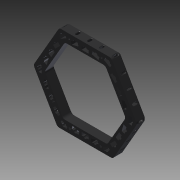
# Autodesk Inventor part: TSOP Cover Ring
Saved by Autodesk Inventor 2015 (Build 190159000, 159)
## iProperties
Created: 2016-10-13
Part Number: TSOP Cover Ring
Material: Generic
Document SubType Name: Modeling
Designer: James Yelland
Density: 1 g/cm^3
Appearance: Default
Author: James Yelland
Autodesk Inventor part; units mm, degrees
ref_plane "YZ Plane" through (0, 0, 0) normal (1, 0, 0) x (0, 1, 0)
ref_plane "XZ Plane" through (0, 0, 0) normal (0, 1, 0) x (-1, 0, 0)
ref_plane "XY Plane" through (0, 0, 0) normal (0, 0, 1) x (1, 0, 0)
sketch "Sketch1" plane through (0, 0, 0) normal (0, 1, 0) x (-1, 0, 0)
  circle A0 centre (24, -57.282) radius 1.6
  circle A1 centre (-25, 62.282) radius 1.6
  circle A2 centre (25, 62.282) radius 1.6
  circle A3 centre (-24, -57.282) radius 1.6
  line L0 (-40, -64.282) -> (40, -64.282)
  arc A4 (40, -64.282) -> (44.3301, -61.782) centre (40, -59.282) ccw
  line L1 (44.3301, -61.782) -> (78.5566, -2.5)
  arc A5 (78.5566, -2.5) -> (78.5566, 2.5) centre (74.2265, 0) ccw
  line L2 (78.5566, 2.5) -> (41.4434, 66.782)
  arc A6 (41.4434, 66.782) -> (37.1132, 69.282) centre (37.1132, 64.282) ccw
  line L3 (37.1132, 69.282) -> (-37.1132, 69.282)
  arc A7 (-37.1132, 69.282) -> (-41.4434, 66.782) centre (-37.1132, 64.282) ccw
  line L4 (-41.4434, 66.782) -> (-78.5566, 2.5)
  arc A8 (-78.5566, 2.5) -> (-78.5566, -2.5) centre (-74.2265, 0) ccw
  line L5 (-78.5566, -2.5) -> (-44.3301, -61.782)
  arc A9 (-44.3301, -61.782) -> (-40, -64.282) centre (-40, -59.282) ccw
  line L6 (47.0096, -27.141) -> (35.6699, -46.782)
  line L7 (0, -49.282) -> (-31.3397, -49.282)
  line L8 (-47.0096, -27.141) -> (-61.2361, -2.5)
  line L9 (-47.0096, 27.141) -> (-32.7831, 51.782)
  line L10 (47.0096, 27.141) -> (32.7831, 51.782)
  line L11 (47.0096, 27.141) -> (61.2361, 2.5)
  line L12 (28.453, 54.282) -> (0, 54.282)
  line L13 (0, 54.282) -> (-28.453, 54.282)
  line L14 (61.2361, -2.5) -> (47.0096, -27.141)
  line L15 (31.3397, -49.282) -> (0, -49.282)
  line L16 (-35.6699, -46.782) -> (-47.0096, -27.141)
  line L17 (-47.0096, 27.141) -> (-61.2361, 2.5)
  arc A10 (31.3397, -49.282) -> (35.6699, -46.782) centre (31.3397, -44.282) ccw
  arc A11 (-35.6699, -46.782) -> (-31.3397, -49.282) centre (-31.3397, -44.282) ccw
  arc A12 (-61.2361, 2.5) -> (-61.2361, -2.5) centre (-56.906, 0) ccw
  arc A13 (-28.453, 54.282) -> (-32.7831, 51.782) centre (-28.453, 49.282) ccw
  arc A14 (32.7831, 51.782) -> (28.453, 54.282) centre (28.453, 49.282) ccw
  arc A15 (61.2361, -2.5) -> (61.2361, 2.5) centre (56.906, 0) ccw
  line L18 (-52.4809, 24.0645) -> (-47.0809, 33.4176)
  arc A16 (-52.6475, 33.376) -> (-55.2282, 28.9061) centre (-53.1151, 30.666) ccw
  line L19 (-56.6378, 26.4645) -> (-55.2282, 28.9061)
  line L20 (-56.6378, 26.4645) -> (-52.4809, 24.0645)
  line L21 (-47.0809, 33.4176) -> (-51.2378, 35.8176)
  line L22 (-52.6475, 33.376) -> (-51.2378, 35.8176)
  line L23 (-56.4865, 20.726) -> (-61.1229, 21.9683)
  line L24 (-61.8526, 19.2451) -> (-61.1229, 21.9683)
  arc A17 (-61.8526, 19.2451) -> (-63.1885, 14.2596) centre (-61.6029, 16.5065) ccw
  line L25 (-59.2817, 10.294) -> (-56.4865, 20.726)
  line L26 (-63.9182, 11.5363) -> (-63.1885, 14.2596)
  line L27 (-63.9182, 11.5363) -> (-59.2817, 10.294)
  line L28 (-67.4265, 5.4) -> (-72.2265, 5.4)
  line L29 (-72.2265, 2.5807) -> (-72.2265, 5.4)
  arc A18 (-72.2265, 2.5807) -> (-72.2265, -2.5807) centre (-71.2765, 0) ccw
  line L30 (-67.4265, -5.4) -> (-67.4265, 5.4)
  line L31 (-72.2265, -5.4) -> (-72.2265, -2.5807)
  line L32 (-72.2265, -5.4) -> (-67.4265, -5.4)
  line L33 (-59.2817, -10.294) -> (-63.9182, -11.5363)
  line L34 (-63.1885, -14.2596) -> (-63.9182, -11.5363)
  arc A19 (-63.1885, -14.2596) -> (-61.8526, -19.2451) centre (-61.6029, -16.5065) ccw
  line L35 (-56.4865, -20.726) -> (-59.2817, -10.294)
  line L36 (-61.1229, -21.9683) -> (-61.8526, -19.2451)
  line L37 (-61.1229, -21.9683) -> (-56.4865, -20.726)
  line L38 (-52.4809, -24.0645) -> (-56.6378, -26.4645)
  line L39 (-55.2282, -28.9061) -> (-56.6378, -26.4645)
  arc A20 (-55.2282, -28.9061) -> (-52.6475, -33.376) centre (-53.1151, -30.666) ccw
  line L40 (-47.0809, -33.4176) -> (-52.4809, -24.0645)
  line L41 (-51.2378, -35.8176) -> (-52.6475, -33.376)
  line L42 (-51.2378, -35.8176) -> (-47.0809, -33.4176)
  line L43 (-46.1925, -38.5557) -> (-49.5866, -41.9498)
  line L44 (-47.593, -43.9434) -> (-49.5866, -41.9498)
  arc A21 (-47.593, -43.9434) -> (-43.9434, -47.593) centre (-45.0965, -45.0965) ccw
  line L45 (-38.5557, -46.1925) -> (-46.1925, -38.5557)
  line L46 (-41.9498, -49.5866) -> (-43.9434, -47.593)
  line L47 (-41.9498, -49.5866) -> (-38.5557, -46.1925)
  line L48 (-35.8898, -51.3629) -> (-38.2898, -55.5199)
  line L49 (-35.8482, -56.9295) -> (-38.2898, -55.5199)
  arc A22 (-35.8482, -56.9295) -> (-31.3783, -59.5102) centre (-33.1382, -57.3971) ccw
  line L50 (-26.5367, -56.7629) -> (-35.8898, -51.3629)
  line L51 (-28.9367, -60.9199) -> (-31.3783, -59.5102)
  line L52 (-28.9367, -60.9199) -> (-26.5367, -56.7629)
  line L53 (-19.3863, -51.4865) -> (-20.6286, -56.1229)
  line L54 (-17.9053, -56.8526) -> (-20.6286, -56.1229)
  arc A23 (-17.9053, -56.8526) -> (-12.9198, -58.1885) centre (-15.1667, -56.6029) ccw
  line L55 (-8.9543, -54.2817) -> (-19.3863, -51.4865)
  line L56 (-10.1966, -58.9182) -> (-12.9198, -58.1885)
  line L57 (-10.1966, -58.9182) -> (-8.9543, -54.2817)
  line L58 (-5.4, -52.482) -> (-5.4, -57.282)
  line L59 (-2.5807, -57.282) -> (-5.4, -57.282)
  arc A24 (-2.5807, -57.282) -> (2.5807, -57.282) centre (0, -56.332) ccw
  line L60 (5.4, -52.482) -> (-5.4, -52.482)
  line L61 (5.4, -57.282) -> (2.5807, -57.282)
  line L62 (5.4, -57.282) -> (5.4, -52.482)
  line L63 (8.9543, -54.2817) -> (10.1966, -58.9182)
  line L64 (12.9198, -58.1885) -> (10.1966, -58.9182)
  arc A25 (12.9198, -58.1885) -> (17.9053, -56.8526) centre (15.1667, -56.6029) ccw
  line L65 (19.3863, -51.4865) -> (8.9543, -54.2817)
  line L66 (20.6286, -56.1229) -> (17.9053, -56.8526)
  line L67 (20.6286, -56.1229) -> (19.3863, -51.4865)
  line L68 (-205.3728, -147.5875) -> (-202.9728, -151.7445)
  line L69 (-200.5312, -150.3348) -> (-202.9728, -151.7445)
  line L70 (-197.3963, -150.6033) -> (-198.7713, -148.2217)
  arc A26 (-200.5312, -150.3348) -> (-196.0613, -147.7541) centre (-198.7713, -148.2217) ccw
  line L71 (-196.0197, -142.1875) -> (-205.3728, -147.5875)
  line L72 (-193.6197, -146.3445) -> (-196.0613, -147.7541)
  line L73 (-193.6197, -146.3445) -> (-196.0197, -142.1875)
  line L74 (38.5557, -46.1925) -> (41.9498, -49.5866)
  line L75 (43.9434, -47.593) -> (41.9498, -49.5866)
  arc A27 (43.9434, -47.593) -> (47.593, -43.9434) centre (45.0965, -45.0965) ccw
  line L76 (46.1925, -38.5557) -> (38.5557, -46.1925)
  line L77 (49.5866, -41.9498) -> (47.593, -43.9434)
  line L78 (49.5866, -41.9498) -> (46.1925, -38.5557)
  line L79 (47.0809, -33.4176) -> (51.2378, -35.8176)
  line L80 (52.6475, -33.376) -> (51.2378, -35.8176)
  arc A28 (52.6475, -33.376) -> (55.2282, -28.9061) centre (53.1151, -30.666) ccw
  line L81 (52.4809, -24.0645) -> (47.0809, -33.4176)
  line L82 (56.6378, -26.4645) -> (55.2282, -28.9061)
  line L83 (56.6378, -26.4645) -> (52.4809, -24.0645)
  line L84 (56.4865, -20.726) -> (61.1229, -21.9683)
  line L85 (61.8526, -19.2451) -> (61.1229, -21.9683)
  arc A29 (61.8526, -19.2451) -> (63.1885, -14.2596) centre (61.6029, -16.5065) ccw
  line L86 (59.2817, -10.294) -> (56.4865, -20.726)
  line L87 (63.9182, -11.5363) -> (63.1885, -14.2596)
  line L88 (63.9182, -11.5363) -> (59.2817, -10.294)
  line L89 (67.4265, -5.4) -> (72.2265, -5.4)
  line L90 (72.2265, -2.5807) -> (72.2265, -5.4)
  arc A30 (72.2265, -2.5807) -> (72.2265, 2.5807) centre (71.2765, 0) ccw
  line L91 (67.4265, 5.4) -> (67.4265, -5.4)
  line L92 (72.2265, 5.4) -> (72.2265, 2.5807)
  line L93 (72.2265, 5.4) -> (67.4265, 5.4)
  line L94 (59.2817, 10.294) -> (63.9182, 11.5363)
  line L95 (63.1885, 14.2596) -> (63.9182, 11.5363)
  arc A31 (63.1885, 14.2596) -> (61.8526, 19.2451) centre (61.6029, 16.5065) ccw
  line L96 (56.4865, 20.726) -> (59.2817, 10.294)
  line L97 (61.1229, 21.9683) -> (61.8526, 19.2451)
  line L98 (61.1229, 21.9683) -> (56.4865, 20.726)
  line L99 (52.4809, 24.0645) -> (56.6378, 26.4645)
  line L100 (55.2282, 28.9061) -> (56.6378, 26.4645)
  arc A32 (55.2282, 28.9061) -> (52.6475, 33.376) centre (53.1151, 30.666) ccw
  line L101 (47.0809, 33.4176) -> (52.4809, 24.0645)
  line L102 (51.2378, 35.8176) -> (52.6475, 33.376)
  line L103 (51.2378, 35.8176) -> (47.0809, 33.4176)
  line L104 (46.1925, 38.5557) -> (49.5866, 41.9498)
  line L105 (47.593, 43.9434) -> (49.5866, 41.9498)
  arc A33 (47.593, 43.9434) -> (43.9434, 47.593) centre (45.0965, 45.0965) ccw
  line L106 (38.5557, 46.1925) -> (46.1925, 38.5557)
  line L107 (41.9498, 49.5866) -> (43.9434, 47.593)
  line L108 (41.9498, 49.5866) -> (38.5557, 46.1925)
  line L109 (38.3898, 55.6931) -> (40.7898, 59.85)
  line L110 (38.3482, 61.2596) -> (40.7898, 59.85)
  arc A34 (38.3482, 61.2596) -> (33.8783, 63.8403) centre (35.6382, 61.7273) ccw
  line L111 (29.0367, 61.0931) -> (38.3898, 55.6931)
  line L112 (31.4367, 65.25) -> (33.8783, 63.8403)
  line L113 (31.4367, 65.25) -> (29.0367, 61.0931)
  line L114 (20.726, 56.4865) -> (21.9683, 61.1229)
  line L115 (19.2451, 61.8526) -> (21.9683, 61.1229)
  arc A35 (19.2451, 61.8526) -> (14.2596, 63.1885) centre (16.5065, 61.6029) ccw
  line L116 (10.294, 59.2817) -> (20.726, 56.4865)
  line L117 (11.5363, 63.9182) -> (14.2596, 63.1885)
  line L118 (11.5363, 63.9182) -> (10.294, 59.2817)
  line L119 (5.4, 57.482) -> (5.4, 62.282)
  line L120 (2.5807, 62.282) -> (5.4, 62.282)
  arc A36 (2.5807, 62.282) -> (-2.5807, 62.282) centre (0, 61.332) ccw
  line L121 (-5.4, 57.482) -> (5.4, 57.482)
  line L122 (-5.4, 62.282) -> (-2.5807, 62.282)
  line L123 (-5.4, 62.282) -> (-5.4, 57.482)
  line L124 (-10.294, 59.2817) -> (-11.5363, 63.9182)
  line L125 (-14.2596, 63.1885) -> (-11.5363, 63.9182)
  arc A37 (-14.2596, 63.1885) -> (-19.2451, 61.8526) centre (-16.5065, 61.6029) ccw
  line L126 (-20.726, 56.4865) -> (-10.294, 59.2817)
  line L127 (-21.9683, 61.1229) -> (-19.2451, 61.8526)
  line L128 (-21.9683, 61.1229) -> (-20.726, 56.4865)
  line L129 (-29.0367, 61.0931) -> (-31.4367, 65.25)
  line L130 (-33.8783, 63.8403) -> (-31.4367, 65.25)
  arc A38 (-33.8783, 63.8403) -> (-38.3482, 61.2596) centre (-35.6382, 61.7273) ccw
  line L131 (-38.3898, 55.6931) -> (-29.0367, 61.0931)
  line L132 (-40.7898, 59.85) -> (-38.3482, 61.2596)
  line L133 (-40.7898, 59.85) -> (-38.3898, 55.6931)
  line L134 (-38.5557, 46.1925) -> (-41.9498, 49.5866)
  line L135 (-43.9434, 47.593) -> (-41.9498, 49.5866)
  arc A39 (-43.9434, 47.593) -> (-47.593, 43.9434) centre (-45.0965, 45.0965) ccw
  line L136 (-46.1925, 38.5557) -> (-38.5557, 46.1925)
  line L137 (-49.5866, 41.9498) -> (-47.593, 43.9434)
  line L138 (-49.5866, 41.9498) -> (-46.1925, 38.5557)
  line L139 (37.9434, -55.7199) -> (35.8482, -56.9295)
  arc A40 (31.3783, -59.5102) -> (35.8482, -56.9295) centre (33.1382, -57.3971) ccw
  line L140 (31.3783, -59.5102) -> (29.2831, -60.7199)
  line L141 (29.2831, -60.7199) -> (27.2831, -57.2558)
  line L142 (27.2831, -57.2558) -> (35.9434, -52.2558)
  line L143 (35.9434, -52.2558) -> (37.9434, -55.7199)
  constraints: 288 end point, 74 point on circle, 52 centre point, 12 tangent, 5 equal radius, 4 horizontal
extrude "Extrusion1" add sketch "Sketch1" along normal blind 15 contours A9 L5 A8 L4 A7 L3 A6 L2 A5 L1 A4 L0
sketch "Sketch2" plane through (0, 15, 0) normal (0, 1, 0) x (1, 0, 0)
  arc A0 (35.6699, 46.782) -> (31.3397, 49.282) centre (31.3397, 44.282) ccw projected
  line L0 (35.6699, 46.782) -> (61.2361, 2.5) projected
  arc A1 (61.2361, -2.5) -> (61.2361, 2.5) centre (56.906, 0) ccw projected
  line L1 (61.2361, -2.5) -> (32.7831, -51.782) projected
  arc A2 (28.453, -54.282) -> (32.7831, -51.782) centre (28.453, -49.282) ccw projected
  line L2 (28.453, -54.282) -> (-28.453, -54.282) projected
  arc A3 (-32.7831, -51.782) -> (-28.453, -54.282) centre (-28.453, -49.282) ccw projected
  line L3 (-32.7831, -51.782) -> (-61.2361, -2.5) projected
  arc A4 (-61.2361, 2.5) -> (-61.2361, -2.5) centre (-56.906, 0) ccw projected
  line L4 (-61.2361, 2.5) -> (-35.6699, 46.782) projected
  arc A5 (-31.3397, 49.282) -> (-35.6699, 46.782) centre (-31.3397, 44.282) ccw projected
  line L5 (-31.3397, 49.282) -> (31.3397, 49.282) projected
  line L6 (38.5557, -46.1925) -> (46.1925, -38.5557) projected
  line L7 (46.1925, -38.5557) -> (49.5866, -41.9498) projected
  line L8 (49.5866, -41.9498) -> (47.593, -43.9434) projected
  arc A6 (43.9434, -47.593) -> (47.593, -43.9434) centre (45.0965, -45.0965) ccw projected
  line L9 (43.9434, -47.593) -> (41.9498, -49.5866) projected
  line L10 (41.9498, -49.5866) -> (38.5557, -46.1925) projected
  line L11 (29.0367, -61.0931) -> (38.3898, -55.6931) projected
  line L12 (38.3898, -55.6931) -> (40.7898, -59.85) projected
  line L13 (40.7898, -59.85) -> (38.3482, -61.2596) projected
  arc A7 (33.8783, -63.8403) -> (38.3482, -61.2596) centre (35.6382, -61.7273) ccw projected
  line L14 (33.8783, -63.8403) -> (31.4367, -65.25) projected
  line L15 (31.4367, -65.25) -> (29.0367, -61.0931) projected
  line L16 (10.294, -59.2817) -> (20.726, -56.4865) projected
  line L17 (20.726, -56.4865) -> (21.9683, -61.1229) projected
  line L18 (21.9683, -61.1229) -> (19.2451, -61.8526) projected
  arc A8 (14.2596, -63.1885) -> (19.2451, -61.8526) centre (16.5065, -61.6029) ccw projected
  line L19 (14.2596, -63.1885) -> (11.5363, -63.9182) projected
  line L20 (11.5363, -63.9182) -> (10.294, -59.2817) projected
  line L21 (-5.4, -57.482) -> (5.4, -57.482) projected
  line L22 (5.4, -57.482) -> (5.4, -62.282) projected
  line L23 (5.4, -62.282) -> (2.5807, -62.282) projected
  arc A9 (-2.5807, -62.282) -> (2.5807, -62.282) centre (0, -61.332) ccw projected
  line L24 (-2.5807, -62.282) -> (-5.4, -62.282) projected
  line L25 (-5.4, -62.282) -> (-5.4, -57.482) projected
  line L26 (-20.726, -56.4865) -> (-10.294, -59.2817) projected
  line L27 (-10.294, -59.2817) -> (-11.5363, -63.9182) projected
  line L28 (-11.5363, -63.9182) -> (-14.2596, -63.1885) projected
  arc A10 (-19.2451, -61.8526) -> (-14.2596, -63.1885) centre (-16.5065, -61.6029) ccw projected
  line L29 (-19.2451, -61.8526) -> (-21.9683, -61.1229) projected
  line L30 (-21.9683, -61.1229) -> (-20.726, -56.4865) projected
  line L31 (-38.3898, -55.6931) -> (-29.0367, -61.0931) projected
  line L32 (-29.0367, -61.0931) -> (-31.4367, -65.25) projected
  line L33 (-31.4367, -65.25) -> (-33.8783, -63.8403) projected
  arc A11 (-38.3482, -61.2596) -> (-33.8783, -63.8403) centre (-35.6382, -61.7273) ccw projected
  line L34 (-38.3482, -61.2596) -> (-40.7898, -59.85) projected
  line L35 (-40.7898, -59.85) -> (-38.3898, -55.6931) projected
  line L36 (-46.1925, -38.5557) -> (-38.5557, -46.1925) projected
  line L37 (-38.5557, -46.1925) -> (-41.9498, -49.5866) projected
  line L38 (-41.9498, -49.5866) -> (-43.9434, -47.593) projected
  arc A12 (-47.593, -43.9434) -> (-43.9434, -47.593) centre (-45.0965, -45.0965) ccw projected
  line L39 (-47.593, -43.9434) -> (-49.5866, -41.9498) projected
  line L40 (-49.5866, -41.9498) -> (-46.1925, -38.5557) projected
  line L41 (-52.4809, -24.0645) -> (-47.0809, -33.4176) projected
  line L42 (-47.0809, -33.4176) -> (-51.2378, -35.8176) projected
  line L43 (-51.2378, -35.8176) -> (-52.6475, -33.376) projected
  arc A13 (-55.2282, -28.9061) -> (-52.6475, -33.376) centre (-53.1151, -30.666) ccw projected
  line L44 (-55.2282, -28.9061) -> (-56.6378, -26.4645) projected
  line L45 (-56.6378, -26.4645) -> (-52.4809, -24.0645) projected
  line L46 (-59.2817, -10.294) -> (-56.4865, -20.726) projected
  line L47 (-56.4865, -20.726) -> (-61.1229, -21.9683) projected
  line L48 (-61.1229, -21.9683) -> (-61.8526, -19.2451) projected
  arc A14 (-63.1885, -14.2596) -> (-61.8526, -19.2451) centre (-61.6029, -16.5065) ccw projected
  line L49 (-63.1885, -14.2596) -> (-63.9182, -11.5363) projected
  line L50 (-63.9182, -11.5363) -> (-59.2817, -10.294) projected
  line L51 (-67.4265, 5.4) -> (-67.4265, -5.4) projected
  line L52 (-67.4265, -5.4) -> (-72.2265, -5.4) projected
  line L53 (-72.2265, -5.4) -> (-72.2265, -2.5807) projected
  arc A15 (-72.2265, 2.5807) -> (-72.2265, -2.5807) centre (-71.2765, 0) ccw projected
  line L54 (-72.2265, 2.5807) -> (-72.2265, 5.4) projected
  line L55 (-72.2265, 5.4) -> (-67.4265, 5.4) projected
  line L56 (-56.4865, 20.726) -> (-59.2817, 10.294) projected
  line L57 (-59.2817, 10.294) -> (-63.9182, 11.5363) projected
  line L58 (-63.9182, 11.5363) -> (-63.1885, 14.2596) projected
  arc A16 (-61.8526, 19.2451) -> (-63.1885, 14.2596) centre (-61.6029, 16.5065) ccw projected
  line L59 (-61.8526, 19.2451) -> (-61.1229, 21.9683) projected
  line L60 (-61.1229, 21.9683) -> (-56.4865, 20.726) projected
  line L61 (-47.0809, 33.4176) -> (-52.4809, 24.0645) projected
  line L62 (-52.4809, 24.0645) -> (-56.6378, 26.4645) projected
  line L63 (-56.6378, 26.4645) -> (-55.2282, 28.9061) projected
  arc A17 (-52.6475, 33.376) -> (-55.2282, 28.9061) centre (-53.1151, 30.666) ccw projected
  line L64 (-52.6475, 33.376) -> (-51.2378, 35.8176) projected
  line L65 (-51.2378, 35.8176) -> (-47.0809, 33.4176) projected
  line L66 (-38.5557, 46.1925) -> (-46.1925, 38.5557) projected
  line L67 (-46.1925, 38.5557) -> (-49.5866, 41.9498) projected
  line L68 (-49.5866, 41.9498) -> (-47.593, 43.9434) projected
  arc A18 (-43.9434, 47.593) -> (-47.593, 43.9434) centre (-45.0965, 45.0965) ccw projected
  line L69 (-43.9434, 47.593) -> (-41.9498, 49.5866) projected
  line L70 (-41.9498, 49.5866) -> (-38.5557, 46.1925) projected
  line L71 (-8.9543, 54.2817) -> (-19.3863, 51.4865) projected
  line L72 (-19.3863, 51.4865) -> (-20.6286, 56.1229) projected
  line L73 (-20.6286, 56.1229) -> (-17.9053, 56.8526) projected
  arc A19 (-12.9198, 58.1885) -> (-17.9053, 56.8526) centre (-15.1667, 56.6029) ccw projected
  line L74 (-12.9198, 58.1885) -> (-10.1966, 58.9182) projected
  line L75 (-10.1966, 58.9182) -> (-8.9543, 54.2817) projected
  line L76 (5.4, 52.482) -> (-5.4, 52.482) projected
  line L77 (-5.4, 52.482) -> (-5.4, 57.282) projected
  line L78 (-5.4, 57.282) -> (-2.5807, 57.282) projected
  arc A20 (2.5807, 57.282) -> (-2.5807, 57.282) centre (0, 56.332) ccw projected
  line L79 (2.5807, 57.282) -> (5.4, 57.282) projected
  line L80 (5.4, 57.282) -> (5.4, 52.482) projected
  line L81 (19.3863, 51.4865) -> (8.9543, 54.2817) projected
  line L82 (8.9543, 54.2817) -> (10.1966, 58.9182) projected
  line L83 (10.1966, 58.9182) -> (12.9198, 58.1885) projected
  arc A21 (17.9053, 56.8526) -> (12.9198, 58.1885) centre (15.1667, 56.6029) ccw projected
  line L84 (17.9053, 56.8526) -> (20.6286, 56.1229) projected
  line L85 (20.6286, 56.1229) -> (19.3863, 51.4865) projected
  line L86 (35.8898, 51.3629) -> (26.5367, 56.7629) projected
  line L87 (26.5367, 56.7629) -> (28.9367, 60.9199) projected
  line L88 (28.9367, 60.9199) -> (31.3783, 59.5102) projected
  arc A22 (35.8482, 56.9295) -> (31.3783, 59.5102) centre (33.1382, 57.3971) ccw projected
  line L89 (35.8482, 56.9295) -> (38.2898, 55.5199) projected
  line L90 (38.2898, 55.5199) -> (35.8898, 51.3629) projected
  line L91 (46.1925, 38.5557) -> (38.5557, 46.1925) projected
  line L92 (38.5557, 46.1925) -> (41.9498, 49.5866) projected
  line L93 (41.9498, 49.5866) -> (43.9434, 47.593) projected
  arc A23 (47.593, 43.9434) -> (43.9434, 47.593) centre (45.0965, 45.0965) ccw projected
  line L94 (47.593, 43.9434) -> (49.5866, 41.9498) projected
  line L95 (49.5866, 41.9498) -> (46.1925, 38.5557) projected
  line L96 (52.4809, 24.0645) -> (47.0809, 33.4176) projected
  line L97 (47.0809, 33.4176) -> (51.2378, 35.8176) projected
  line L98 (51.2378, 35.8176) -> (52.6475, 33.376) projected
  arc A24 (55.2282, 28.9061) -> (52.6475, 33.376) centre (53.1151, 30.666) ccw projected
  line L99 (55.2282, 28.9061) -> (56.6378, 26.4645) projected
  line L100 (56.6378, 26.4645) -> (52.4809, 24.0645) projected
  line L101 (59.2817, 10.294) -> (56.4865, 20.726) projected
  line L102 (56.4865, 20.726) -> (61.1229, 21.9683) projected
  line L103 (61.1229, 21.9683) -> (61.8526, 19.2451) projected
  arc A25 (63.1885, 14.2596) -> (61.8526, 19.2451) centre (61.6029, 16.5065) ccw projected
  line L104 (63.1885, 14.2596) -> (63.9182, 11.5363) projected
  line L105 (63.9182, 11.5363) -> (59.2817, 10.294) projected
  line L106 (67.4265, -5.4) -> (67.4265, 5.4) projected
  line L107 (67.4265, 5.4) -> (72.2265, 5.4) projected
  line L108 (72.2265, 5.4) -> (72.2265, 2.5807) projected
  arc A26 (72.2265, -2.5807) -> (72.2265, 2.5807) centre (71.2765, 0) ccw projected
  line L109 (72.2265, -2.5807) -> (72.2265, -5.4) projected
  line L110 (72.2265, -5.4) -> (67.4265, -5.4) projected
  line L111 (56.4865, -20.726) -> (59.2817, -10.294) projected
  line L112 (59.2817, -10.294) -> (63.9182, -11.5363) projected
  line L113 (63.9182, -11.5363) -> (63.1885, -14.2596) projected
  arc A27 (61.8526, -19.2451) -> (63.1885, -14.2596) centre (61.6029, -16.5065) ccw projected
  line L114 (61.8526, -19.2451) -> (61.1229, -21.9683) projected
  line L115 (61.1229, -21.9683) -> (56.4865, -20.726) projected
  line L116 (52.4809, -24.0645) -> (56.6378, -26.4645) projected
  line L117 (56.6378, -26.4645) -> (55.2282, -28.9061) projected
  arc A28 (52.6475, -33.376) -> (55.2282, -28.9061) centre (53.1151, -30.666) ccw projected
  line L118 (52.6475, -33.376) -> (51.2378, -35.8176) projected
  line L119 (51.2378, -35.8176) -> (47.0809, -33.4176) projected
  line L120 (47.0809, -33.4176) -> (52.4809, -24.0645) projected
  line L121 (-27.2831, 57.2558) -> (-35.9434, 52.2558) projected
  line L122 (-35.9434, 52.2558) -> (-37.9434, 55.7199) projected
  line L123 (-37.9434, 55.7199) -> (-35.8482, 56.9295) projected
  arc A29 (-31.3783, 59.5102) -> (-35.8482, 56.9295) centre (-33.1382, 57.3971) ccw projected
  line L124 (-31.3783, 59.5102) -> (-29.2831, 60.7199) projected
  line L125 (-29.2831, 60.7199) -> (-27.2831, 57.2558) projected
  circle A30 centre (-25, -62.282) radius 1.6 projected
  circle A31 centre (24, 57.282) radius 1.6 projected
  circle A32 centre (25, -62.282) radius 1.6 projected
  circle A33 centre (-24, 57.282) radius 1.6 projected
  line L126 (40, 64.282) -> (-40, 64.282) projected
  arc A34 (-40, 64.282) -> (-44.3301, 61.782) centre (-40, 59.282) ccw projected
  line L127 (-44.3301, 61.782) -> (-78.5566, 2.5) projected
  arc A35 (-78.5566, 2.5) -> (-78.5566, -2.5) centre (-74.2265, 0) ccw projected
  line L128 (-78.5566, -2.5) -> (-41.4434, -66.782) projected
  arc A36 (-41.4434, -66.782) -> (-37.1132, -69.282) centre (-37.1132, -64.282) ccw projected
  line L129 (-37.1132, -69.282) -> (37.1132, -69.282) projected
  arc A37 (37.1132, -69.282) -> (41.4434, -66.782) centre (37.1132, -64.282) ccw projected
  line L130 (41.4434, -66.782) -> (78.5566, -2.5) projected
  arc A38 (78.5566, -2.5) -> (78.5566, 2.5) centre (74.2265, 0) ccw projected
  line L131 (78.5566, 2.5) -> (44.3301, 61.782) projected
  arc A39 (44.3301, 61.782) -> (40, 64.282) centre (40, 59.282) ccw projected
  point P0 (0, 0)
extrude "Extrusion2" add sketch "Sketch2" against normal blind 2 contours L6 L7 L8 A6 L9 L10 | L11 L12 L13 A7 L14 L15 | L16 L17 L18 A8 L19 L20 | L21 L22 L23 A9 L24 L25 | L26 L27 L28 A10 L29 L30 | L31 L32 L33 A11 L34 L35 | L36 L37 L38 A12 L39 L40 | L41 L42 L43 A13 L44 L45 | L46 L47 L48 A14 L49 L50 | L51 L52 L53 A15 L54 L55 | L56 L57 L58 A16 L59 L60 | L61 L62 L63 A17 L64 L65 | L66 L67 L68 A18 L69 L70 | L71 L72 L73 A19 L74 L75 | L76 L77 L78 A20 L79 L80 | L81 L82 L83 A21 L84 L85 | L86 L87 L88 A22 L89 L90 | L91 L92 L93 A23 L94 L95 | L96 L97 L98 A24 L99 L100 | L101 L102 L103 A25 L104 L105 | L106 L107 L108 A26 L109 L110 | L111 L112 L113 A27 L114 L115 | L116 L117 A28 L118 L119 L120 | L121 L122 L123 A29 L124 L125
chamfer "Chamfer1" distance 2 angle 45 12 edges at (0, 15, 69.282) (39.6132, 15, 68.6122) (60, 15, 34.641) (79.2265, 15, 0) (61.4434, 15, -32.141) (42.5, 15, -63.6122) (0, 15, -64.282) (-42.5, 15, -63.6122) (-61.4434, 15, -32.141) (-79.2265, 15, 0) (-60, 15, 34.641) (-39.6132, 15, 68.6122)
sketch "Sketch3" plane through (-47.0809, 0, -33.4176) normal (-0.8660254, 0, -0.5) x (-0.5, 0, 0.8660254)
  line L0 (5.4, 0) -> (5.4, 9.5)
  line L1 (3.9, 9.5) -> (3.9, 5.5)
  line L2 (6.9, 9.5) -> (6.9, 5.5)
  arc A0 (6.9, 9.5) -> (3.9, 9.5) centre (5.4, 9.5) ccw
  arc A1 (3.9, 5.5) -> (6.9, 5.5) centre (5.4, 5.5) ccw
  dimension "d27" = 9.5
  dimension "d29" = 4
  dimension "d30" = 4
  constraints: 6 end point, 4 point on circle, 3 vertical, 2 centre point, 1 coincident, 1 point on line
  measures "d27" distance of L0.start L0.end
  measures "d29" distance of L1.start L1.end
  measures "d30" distance of L2.start L2.end
extrude "Extrusion3" cut sketch "Sketch3" along normal through all
pattern_circular "Circular Pattern1" count 5 over 240 about axis through (0, -10, 0) along (0, 1, 0) of "Extrusion3"
sketch "Sketch4" plane through (46.1925, 0, -38.5557) normal (0.7071068, 0, -0.7071068) x (-0.7071068, 0, -0.7071068)
  line L0 (5.4, 0) -> (5.4, 9.5)
  line L1 (3.9, 9.5) -> (3.9, 5.5)
  line L2 (6.9, 9.5) -> (6.9, 5.5)
  arc A0 (6.9, 9.5) -> (3.9, 9.5) centre (5.4, 9.5) ccw
  arc A1 (3.9, 5.5) -> (6.9, 5.5) centre (5.4, 5.5) ccw
  point P0 (5.4, 0)
  dimension "d39" = 9.5
  dimension "d40" = 4
  dimension "d41" = 4
  constraints: 6 end point, 4 point on circle, 3 vertical, 2 centre point, 1 coincident, 1 point on line
  measures "d39" distance of L0.start L0.end
  measures "d40" distance of L1.start L1.end
  measures "d41" distance of L2.start L2.end
extrude "Extrusion4" cut sketch "Sketch4" along normal through all
pattern_circular "Circular Pattern2" count 5 over 240 about axis through (0, -10, 0) along (0, -1, 0) of "Extrusion4"
sketch "Sketch5" plane through (59.2817, 0, -10.294) normal (0.9659258, 0, -0.258819) x (-0.258819, 0, -0.9659258)
  line L0 (5.4, 0) -> (5.4, 9.5)
  line L1 (3.9, 9.5) -> (3.9, 5.5)
  line L2 (6.9, 9.5) -> (6.9, 5.5)
  arc A0 (6.9, 9.5) -> (3.9, 9.5) centre (5.4, 9.5) ccw
  arc A1 (3.9, 5.5) -> (6.9, 5.5) centre (5.4, 5.5) ccw
  point P0 (5.4, 0)
  dimension "d47" = 9.5
  dimension "d48" = 4
  dimension "d49" = 4
  constraints: 6 end point, 4 point on circle, 3 vertical, 2 centre point, 1 coincident, 1 point on line
  measures "d47" distance of L0.start L0.end
  measures "d48" distance of L1.start L1.end
  measures "d49" distance of L2.start L2.end
extrude "Extrusion5" cut sketch "Sketch5" along normal through all
pattern_circular "Circular Pattern3" count 5 over 240 about axis through (0, -10, 0) along (0, -1, 0) of "Extrusion5"
sketch "Sketch6" plane through (67.4265, 0, 5.4) normal (1, 0, 0) x (0, 0, -1)
  line L0 (5.4, 0) -> (5.4, 9.5)
  line L1 (3.9, 9.5) -> (3.9, 5.5)
  line L2 (6.9, 9.5) -> (6.9, 5.5)
  arc A0 (6.9, 9.5) -> (3.9, 9.5) centre (5.4, 9.5) ccw
  arc A1 (3.9, 5.5) -> (6.9, 5.5) centre (5.4, 5.5) ccw
  point P0 (5.4, 0)
  dimension "d55" = 9.5
  dimension "d56" = 4
  dimension "d57" = 4
  constraints: 6 end point, 4 point on circle, 3 vertical, 2 centre point, 1 coincident, 1 point on line
  measures "d55" distance of L0.start L0.end
  measures "d56" distance of L1.start L1.end
  measures "d57" distance of L2.start L2.end
extrude "Extrusion6" cut sketch "Sketch6" along normal through all
pattern_circular "Circular Pattern4" count 4 over 180 about axis through (0, -10, 0) along (0, -1, 0) of "Extrusion6"
sketch "Sketch7" plane through (35.8898, 0, -51.3629) normal (0.5, 0, -0.8660254) x (-0.8660254, 0, -0.5)
  line L0 (5.4, 0) -> (5.4, 9.5)
  line L1 (3.9, 9.5) -> (3.9, 5.5)
  line L2 (6.9, 9.5) -> (6.9, 5.5)
  arc A0 (6.9, 9.5) -> (3.9, 9.5) centre (5.4, 9.5) ccw
  arc A1 (3.9, 5.5) -> (6.9, 5.5) centre (5.4, 5.5) ccw
  point P0 (5.4, 0)
  dimension "d63" = 9.5
  dimension "d64" = 4
  dimension "d65" = 4
  constraints: 6 end point, 4 point on circle, 3 vertical, 2 centre point, 1 coincident, 1 point on line
  measures "d63" distance of L0.start L0.end
  measures "d64" distance of L1.start L1.end
  measures "d65" distance of L2.start L2.end
sketch "Sketch8" plane through (19.3863, 0, -51.4865) normal (0.258819, 0, -0.9659258) x (-0.9659258, 0, -0.258819)
  line L0 (5.4, 0) -> (5.4, 9.5)
  line L1 (3.9, 9.5) -> (3.9, 5.5)
  line L2 (6.9, 9.5) -> (6.9, 5.5)
  arc A0 (6.9, 9.5) -> (3.9, 9.5) centre (5.4, 9.5) ccw
  arc A1 (3.9, 5.5) -> (6.9, 5.5) centre (5.4, 5.5) ccw
  point P0 (5.4, 0)
  dimension "d66" = 9.5
  dimension "d67" = 4
  dimension "d68" = 4
  constraints: 6 end point, 4 point on circle, 3 vertical, 2 centre point, 1 coincident, 1 point on line
  measures "d66" distance of L0.start L0.end
  measures "d67" distance of L1.start L1.end
  measures "d68" distance of L2.start L2.end
sketch "Sketch9" plane through (5.4, 0, -52.482) normal (0, 0, -1) x (-1, 0, 0)
  line L0 (5.4, 0) -> (5.4, 9.5)
  line L1 (3.9, 9.5) -> (3.9, 5.5)
  line L2 (6.9, 9.5) -> (6.9, 5.5)
  arc A0 (6.9, 9.5) -> (3.9, 9.5) centre (5.4, 9.5) ccw
  arc A1 (3.9, 5.5) -> (6.9, 5.5) centre (5.4, 5.5) ccw
  point P0 (5.4, 0)
  dimension "d69" = 9.5
  dimension "d70" = 4
  dimension "d71" = 4
  constraints: 6 end point, 4 point on circle, 3 vertical, 2 centre point, 1 coincident, 1 point on line
  measures "d69" distance of L0.start L0.end
  measures "d70" distance of L1.start L1.end
  measures "d71" distance of L2.start L2.end
sketch "Sketch10" plane through (-8.9543, 0, -54.2817) normal (-0.258819, 0, -0.9659258) x (-0.9659258, 0, 0.258819)
  line L0 (5.4, 0) -> (5.4, 9.5)
  line L1 (3.9, 9.5) -> (3.9, 5.5)
  line L2 (6.9, 9.5) -> (6.9, 5.5)
  arc A0 (6.9, 9.5) -> (3.9, 9.5) centre (5.4, 9.5) ccw
  arc A1 (3.9, 5.5) -> (6.9, 5.5) centre (5.4, 5.5) ccw
  point P0 (5.4, 0)
  dimension "d72" = 9.5
  dimension "d73" = 4
  dimension "d74" = 4
  constraints: 6 end point, 4 point on circle, 3 vertical, 2 centre point, 1 coincident, 1 point on line
  measures "d72" distance of L0.start L0.end
  measures "d73" distance of L1.start L1.end
  measures "d74" distance of L2.start L2.end
sketch "Sketch11" plane through (-27.2831, 0, -57.2558) normal (-0.5, 0, -0.8660254) x (-0.8660254, 0, 0.5)
  line L0 (5.4, 0) -> (5.4, 9.5)
  line L1 (3.9, 9.5) -> (3.9, 5.5)
  line L2 (6.9, 9.5) -> (6.9, 5.5)
  arc A0 (6.9, 9.5) -> (3.9, 9.5) centre (5.4, 9.5) ccw
  arc A1 (3.9, 5.5) -> (6.9, 5.5) centre (5.4, 5.5) ccw
  point P0 (5, 0)
  dimension "d75" = 9.5
  dimension "d76" = 4
  dimension "d77" = 4
  constraints: 6 end point, 4 point on circle, 3 vertical, 2 centre point, 1 coincident, 1 point on line
  measures "d75" distance of L0.start L0.end
  measures "d76" distance of L1.start L1.end
  measures "d77" distance of L2.start L2.end
extrude "Extrusion7" cut sketch "Sketch11" along normal through all
extrude "Extrusion8" cut sketch "Sketch10" along normal through all
extrude "Extrusion9" cut sketch "Sketch9" along normal through all
extrude "Extrusion10" cut sketch "Sketch8" along normal through all
extrude "Extrusion11" cut sketch "Sketch7" along normal through all
chamfer "Chamfer3" distance 0.5 angle 45 96 edges at (35.3812, 7.5, -64.282) (37.1132, 4, -64.282) (38.8453, 7.5, -64.282) (37.1132, 11, -64.282) (18.7772, 7.5, -64.282) (17.2243, 11, -64.282) (15.6714, 7.5, -64.282) (17.2243, 4, -64.282) (1.5, 7.5, -64.282) (0, 11, -64.282) (-1.5, 7.5, -64.282) (0, 4, -64.282) (-15.6714, 7.5, -64.282) (-17.2243, 11, -64.282) (-18.7772, 7.5, -64.282) (-17.2243, 4, -64.282) (-39.3072, 7.5, -64.282) (-37.5751, 4, -64.282) (-35.8431, 7.5, -64.282) (-37.5751, 11, -64.282) (-51.4944, 7.5, -49.3731) (-50.718, 4, -50.718) (-49.9415, 7.5, -52.0628) (-50.718, 11, -50.718) (-60.75, 7.5, -33.342) (-60, 4, -34.641) (-59.25, 7.5, -35.9401) (-60, 11, -34.641) (-70.0585, 7.5, -17.2192) (-69.282, 4, -18.5641) (-68.5056, 7.5, -19.9089) (-69.282, 11, -18.5641) (-79.2265, 11, 0.0021) (-78.9962, 7.5, 1.5) (-79.2265, 4, 0.0034) (-78.9962, 7.5, -1.5) (-69.282, 11, 18.5641) (-68.5056, 7.5, 19.9089) (-69.282, 4, 18.5641) (-70.0585, 7.5, 17.2192) (-60, 11, 34.641) (-59.25, 7.5, 35.9401) (-60, 4, 34.641) (-60.75, 7.5, 33.342) (-49.9415, 7.5, 52.0628) (-50.718, 4, 50.718) (-51.4944, 7.5, 49.3731) (-50.718, 11, 50.718) (-40.7971, 7.5, 67.6627) (-39.6115, 11, 68.6132) (-38.1991, 7.5, 69.1627) (-39.6103, 4, 68.6139) (1.5, 7.5, 69.282) (0, 4, 69.282) (-1.5, 7.5, 69.282) (0, 11, 69.282) (17.0112, 7.5, 69.282) (18.5641, 11, 69.282) (20.117, 7.5, 69.282) (18.5641, 4, 69.282) (38.1991, 7.5, 69.1627) (39.615, 11, 68.6111) (40.7971, 7.5, 67.6627) (39.6162, 4, 68.6104) (-18.5641, 4, 69.282) (-20.117, 7.5, 69.282) (-18.5641, 11, 69.282) (-17.0112, 7.5, 69.282) (49.9415, 7.5, 52.0628) (50.718, 11, 50.718) (51.4944, 7.5, 49.3731) (50.718, 4, 50.718) (60.75, 7.5, 33.342) (60, 4, 34.641) (59.25, 7.5, 35.9401) (60, 11, 34.641) (68.5056, 7.5, 19.9089) (69.282, 11, 18.5641) (70.0585, 7.5, 17.2192) (69.282, 4, 18.5641) (78.9962, 7.5, 1.5) (79.2265, 11, -0.0021) (78.9962, 7.5, -1.5) (79.2231, 4.0113, 0.1834) (70.0585, 7.5, -17.2192) (69.282, 11, -18.5641) (68.5056, 7.5, -19.9089) (69.282, 4, -18.5641) (60.75, 7.5, -33.342) (60, 11, -34.641) (59.25, 7.5, -35.9401) (60, 4, -34.641) (51.4944, 7.5, -49.3731) (50.718, 11, -50.718) (49.9415, 7.5, -52.0628) (50.718, 4, -50.718)
chamfer "Chamfer4" distance 2 angle 45 12 edges at (47.0096, 15, 27.141) (30.953, 15, 53.6122) (0, 15, 54.282) (-30.953, 15, 53.6122) (-47.0096, 15, 27.141) (-61.906, 15, 0) (-48.453, 15, -24.641) (-33.8397, 15, -48.6122) (0, 15, -49.282) (33.8397, 15, -48.6122) (48.453, 15, -24.641) (61.906, 15, 0)
body "Solid1"
